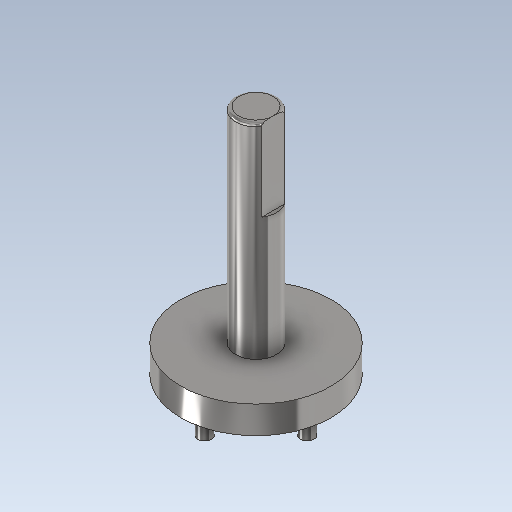
# Autodesk Inventor part: 555_GearBox_Shaft
Saved by Autodesk Inventor 2021 (Build 250183000, 183)
## iProperties
Created: 2021-08-07
Part Number: 555_GearBox_Shaft
Material: 鉄、鋳鉄
Document SubType Name: Modeling
Designer: Hagihara Yuya
Density: 7.15 g/cm^3
Appearance: 鋼 - つや出し
Author: Hagihara Yuya
Autodesk Inventor part; units mm, degrees
ref_plane "YZ Plane" through (0, 0, 0) normal (1, 0, 0) x (0, 1, 0)
ref_plane "XZ Plane" through (0, 0, 0) normal (0, 1, 0) x (-1, 0, 0)
ref_plane "XY Plane" through (0, 0, 0) normal (0, 0, 1) x (1, 0, 0)
sketch "スケッチ1" plane through (0, 0, 0) normal (0, 0, 1) x (1, 0, 0)
  circle A0 centre (0, 0) radius 11
  dimension "d0" = 22
  constraints: 1 centre point, 1 coincident
  measures "d0" diameter of A0
extrude "押し出し1" add sketch "スケッチ1" along normal blind 4
sketch "スケッチ2" plane through (0, 0, 4) normal (0, 0, 1) x (1, 0, 0)
  circle A0 centre (0, 0) radius 11 projected
  circle A1 centre (0, 0) radius 3
  dimension "d3" = 6
  constraints: 1 centre point, 1 coincident
  measures "d3" diameter of A1
extrude "押し出し2" add sketch "スケッチ2" along normal blind 30 contours A1
sketch "スケッチ3" plane through (0, 0, 0) normal (0, 0, -1) x (-1, 0, 0)
  circle A0 centre (0, 7.5) radius 1
  circle A1 centre (-7.5, 0) radius 1
  circle A2 centre (0, -7.5) radius 1
  circle A3 centre (7.5, 0) radius 1
  point P0 (0, 0)
  dimension "d6" = 2
  dimension "d7" = 7.5
  dimension "d10" = 360
  constraints: 4 centre point, 1 vertical alignment, 9 other
  measures "d6" diameter of A0
  measures "d7" distance of point (0, 0) A0.centre
extrude "押し出し3" add sketch "スケッチ3" along normal blind 4
fillet "フィレット1" radius 0.5 1 edges at (-3, 0, 34)
sketch "スケッチ4" plane through (0, 0, 34) normal (0, 0, 1) x (1, 0, 0)
  line L0 (-3, -1.6583) -> (-2.5, -1.6583)
  line L1 (-2.5, -1.6583) -> (-2.5, 1.6583)
  line L2 (-2.5, 1.6583) -> (-3, 1.6583)
  line L3 (-3, 1.6583) -> (-3, -1.6583)
  circle A0 centre (0, 0) radius 3 projected
  point P0 (-2.5, 0)
  dimension "d15" = 0.5
  constraints: 8 end point, 2 parallel, 1 horizontal, 1 horizontal alignment, 1 midpoint, 1 perpendicular, 1 vertical, 2 other
  measures "d15" distance of L1.end L2.end
extrude "押し出し4" cut sketch "スケッチ4" against normal blind 12 contours A0 L1 picked at (-2.5914, 0.3806)
